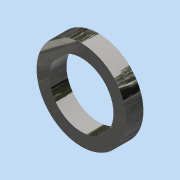
# Autodesk Inventor part: M8Bearing
Saved by Autodesk Inventor 2015 (Build 190159000, 159)
## iProperties
Created: 2015-12-23
Part Number: M8Bearing
Material: Steel, Alloy
Document SubType Name: Modeling
Designer: Raphael
Density: 7.73 g/cm^3
Appearance: Steel - Polished
Title: 7804K115.step
Description: STEP AP203
Creation Date: 2015-09-11
Sending System: SolidWorks 2010
Preprocessor: SwSTEP 2.0
Author: Raphael
Autodesk Inventor part; units mm, degrees
ref_plane "YZ Plane" through (0, 0, 0) normal (1, 0, 0) x (0, 1, 0)
ref_plane "XZ Plane" through (0, 0, 0) normal (0, 1, 0) x (-1, 0, 0)
ref_plane "XY Plane" through (0, 0, 0) normal (0, 0, 1) x (1, 0, 0)
sketch "Sketch1" plane through (0, 0, 0) normal (0, 0, 1) x (1, 0, 0)
  circle A0 centre (0, 0) radius 7.5
  circle A1 centre (0, 0) radius 10.5
  dimension "d0" = 15
  dimension "d1" = 21
  constraints: 2 centre point, 2 coincident
  measures "d0" diameter of A0
  measures "d1" diameter of A1
extrude "Extrusion1" add sketch "Sketch1" along normal mid plane 4
body "Solid17"
